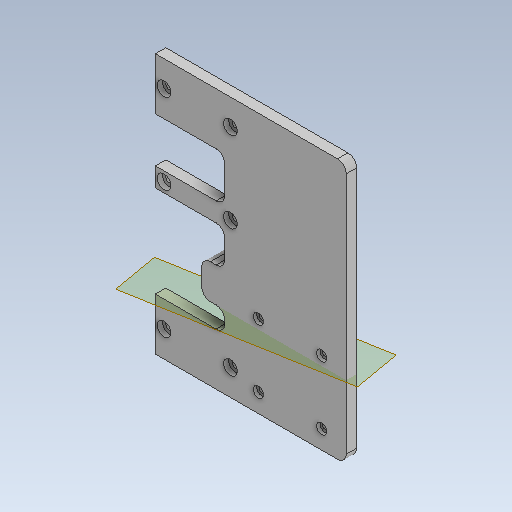
# Autodesk Inventor part: PlacaBase
Saved by Autodesk Inventor 2021 (Build 250183000, 183)
## iProperties
Created: 2022-10-28
Part Number: PlacaBase
Material: Generic
Document SubType Name: Modeling
Designer: zulet
Density: 1 g/cm^3
Appearance: Default
Author: zulet
Autodesk Inventor part; units mm, degrees
ref_plane "YZ Plane" through (0, 0, 0) normal (1, 0, 0) x (0, 1, 0)
ref_plane "XZ Plane" through (0, 0, 0) normal (0, 1, 0) x (-1, 0, 0)
ref_plane "XY Plane" through (0, 0, 0) normal (0, 0, 1) x (1, 0, 0)
sketch "Sketch1" plane through (0, 0, 0) normal (0, 0, 1) x (1, 0, 0)
  line L0 (-40, -150) -> (70, -150)
  line L1 (70, -150) -> (70, 0)
  line L2 (70, 0) -> (-40, 0)
  line L3 (-40, 0) -> (-40, -30)
  line L4 (-40, -30) -> (0, -30)
  line L5 (0, -30) -> (0, -56)
  line L6 (0, -56) -> (-40, -56)
  line L7 (-40, -56) -> (-40, -67)
  line L8 (-40, -67) -> (0, -67)
  line L9 (0, -67) -> (0, -120)
  line L10 (0, -120) -> (-40, -120)
  line L11 (-40, -120) -> (-40, -150)
  circle A0 centre (-35, -15) radius 2
  circle A1 centre (3.24, -15) radius 2
  line L12 (-35, -15) -> (3.24, -15) construction
  line L13 (-35, -15) -> (-40, -15) construction
  line L14 (-62, 0) -> (92, 0) projected
  line L15 (0, -180) -> (0, 30) projected
  circle A2 centre (-35, -61.5) radius 2
  circle A3 centre (3.24, -61.5) radius 2
  line L16 (-35, -61.5) -> (3.24, -61.5) construction
  circle A4 centre (-35, -135) radius 2
  line L17 (-35, -135) -> (3.24, -135) construction
  circle A5 centre (3.24, -135) radius 2
  line L18 (9.12, -7) -> (66.12, -7)
  line L19 (66.12, -7) -> (66.12, -92)
  line L20 (66.12, -92) -> (9.12, -92)
  line L21 (9.12, -92) -> (9.12, -7)
  line L22 (15.62, -99) -> (59.62, -99)
  line L23 (59.62, -99) -> (59.62, -143)
  line L24 (59.62, -143) -> (15.62, -143)
  line L25 (15.62, -143) -> (15.62, -99)
  line L26 (15.62, -99) -> (59.62, -143) construction
  line L27 (15.62, -143) -> (59.62, -99) construction
  circle A6 centre (19.37, -102.75) radius 1.5
  circle A7 centre (19.37, -139.25) radius 1.5
  circle A8 centre (55.87, -139.25) radius 1.5
  circle A9 centre (55.87, -102.75) radius 1.5
  line L28 (19.37, -102.75) -> (19.37, -139.25) construction
  line L29 (19.37, -139.25) -> (55.87, -139.25) construction
  line L30 (55.87, -139.25) -> (55.87, -102.75) construction
  line L31 (55.87, -102.75) -> (19.37, -102.75) construction
  line L32 (37.62, -7) -> (37.62, -92) construction
  line L33 (37.62, -99) -> (37.62, -143) construction
  point P0 (0, 0)
  dimension "d2" = 4
  dimension "d3" = 4
  dimension "d4" = 38.24
  dimension "d5" = 5
  dimension "d6" = 30
  dimension "d7" = 11
  dimension "d8" = 30
  dimension "d11" = 46.5
  dimension "d18" = 46.5
  dimension "d25" = 120
  dimension "d30" = 57
  dimension "d31" = 85
  dimension "d32" = 44
  dimension "d33" = 44
  dimension "d34" = 40
  dimension "d35" = 70
  dimension "d36" = 3
  dimension "d37" = 3
  dimension "d38" = 3
  dimension "d39" = 3
  dimension "d40" = 36.5
  dimension "d42" = 7
  dimension "d43" = 7
  dimension "d44" = 7
  dimension "d45" = 3.88
  dimension "d46" = 3.88
  constraints: 64 end point, 13 perpendicular, 10 centre point, 9 point on line, 6 horizontal, 5 midpoint, 4 collinear, 4 parallel, 4 vertical, 14 other
  measures "d2" diameter of A0
  measures "d3" diameter of A1
  measures "d4" distance of L12.start L12.end
  measures "d5" distance of L12.start L13.end
  measures "d6" distance between parallel lines of L4 L2
  measures "d7" distance between parallel lines of L8 L6
  measures "d8" distance between parallel lines of L0 L10
  measures "d11" distance of L12.start A2.centre
  measures "d18" distance of L12.start L16.start
  measures "d25" distance of L12.start L17.start
  measures "d30" distance of L19.end L20.end
  measures "d31" distance of L18.end L19.end
  measures "d32" distance of L23.end L24.end
  measures "d33" distance of L22.end L23.end
  measures "d34" distance between parallel lines of L15 L3
  measures "d35" distance between parallel lines of L1 L15
  measures "d36" diameter of A6
  measures "d37" diameter of A7
  measures "d38" diameter of A8
  measures "d39" diameter of A9
  measures "d40" distance of L28.end L28.start
  measures "d42" distance between parallel lines of L18 L14
  measures "d43" distance between parallel lines of L22 L20
  measures "d44" distance between parallel lines of L0 L24
  measures "d45" distance edge to line of A3 L21
  measures "d46" distance between parallel lines of L1 L19
extrude "Extrusion1" add sketch "Sketch1" along normal blind 6 contours L11 L10 L15 L0 | L15 L9 L5 L2 L1 L0 | L8 L7 L6 L15 | L15 L4 L3 L2
sketch "Sketch2" plane through (0, 0, 6) normal (0, 0, 1) x (1, 0, 0)
  line L0 (0, -56) -> (-40, -56) projected
  line L1 (-40, -56) -> (-40, -67) projected
  line L2 (-40, -67) -> (0, -67) projected
  line L3 (0, -67) -> (0, -120) projected
  line L4 (0, -120) -> (-40, -120) projected
  line L5 (-40, -120) -> (-40, -150) projected
  line L6 (-40, -150) -> (70, -150) projected
  line L7 (70, -150) -> (70, 0) projected
  line L8 (70, 0) -> (-40, 0) projected
  line L9 (-40, 0) -> (-40, -30) projected
  line L10 (-40, -30) -> (0, -30) projected
  line L11 (0, -30) -> (0, -56) projected
  circle A0 centre (-35, -15) radius 2 projected
  circle A1 centre (-35, -61.5) radius 2 projected
  circle A2 centre (-35, -135) radius 2 projected
  circle A3 centre (3.24, -15) radius 2 projected
  circle A4 centre (3.24, -61.5) radius 2 projected
  circle A5 centre (3.24, -135) radius 2 projected
  line L12 (15.62, -99) -> (59.62, -99) projected
  line L13 (59.62, -99) -> (59.62, -143) projected
  line L14 (59.62, -143) -> (15.62, -143) projected
  line L15 (15.62, -143) -> (15.62, -99) projected
  line L16 (9.12, -7) -> (66.12, -7) projected
  line L17 (66.12, -7) -> (66.12, -92) projected
  line L18 (66.12, -92) -> (9.12, -92) projected
  line L19 (9.12, -92) -> (9.12, -7) projected
  circle A6 centre (19.37, -102.75) radius 1.5 projected
  circle A7 centre (19.37, -139.25) radius 1.5 projected
  circle A8 centre (55.87, -139.25) radius 1.5 projected
  circle A9 centre (55.87, -102.75) radius 1.5 projected
  point P0 (0, 0)
extrude "Extrusion2" add sketch "Sketch2" against normal blind 3 contours L12 L13 L14 L15 | L16 L17 L18 L19
fillet "Fillet1" radius 5 6 edges at (0, -56, 3) (0, -30, 3) (0, -67, 3) (0, -120, 3) (70, 0, 3) (70, -150, 3)
sketch "Sketch3" plane through (0, 0, 6) normal (0, 0, 1) x (1, 0, 0)
  circle A0 centre (-35, -15) radius 2 projected
  circle A1 centre (-35, -15) radius 4
  circle A2 centre (3.24, -15) radius 2 projected
  circle A3 centre (3.24, -15) radius 4
  circle A4 centre (3.24, -61.5) radius 2 projected
  circle A5 centre (3.24, -61.5) radius 4
  circle A6 centre (-35, -61.5) radius 2 projected
  circle A7 centre (-35, -61.5) radius 4
  circle A8 centre (-35, -135) radius 2 projected
  circle A9 centre (-35, -135) radius 4
  circle A10 centre (3.24, -135) radius 2 projected
  circle A11 centre (3.24, -135) radius 4
  circle A12 centre (55.87, -102.75) radius 1.5 projected
  circle A13 centre (55.87, -102.75) radius 3
  circle A14 centre (55.87, -139.25) radius 1.5 projected
  circle A15 centre (55.87, -139.25) radius 3
  circle A16 centre (19.37, -139.25) radius 1.5 projected
  circle A17 centre (19.37, -139.25) radius 3
  circle A18 centre (19.37, -102.75) radius 1.5 projected
  circle A19 centre (19.37, -102.75) radius 3
  point P0 (0, 0)
  dimension "d50" = 8
  dimension "d51" = 8
  dimension "d52" = 8
  dimension "d53" = 8
  dimension "d54" = 8
  dimension "d55" = 8
  dimension "d58" = 6
  dimension "d59" = 6
  dimension "d60" = 6
  dimension "d61" = 6
  constraints: 10 centre point, 10 coincident
  measures "d50" diameter of A1
  measures "d51" diameter of A3
  measures "d52" diameter of A5
  measures "d53" diameter of A7
  measures "d54" diameter of A9
  measures "d55" diameter of A11
  measures "d58" diameter of A13
  measures "d59" diameter of A15
  measures "d60" diameter of A17
  measures "d61" diameter of A19
extrude "Extrusion3" cut sketch "Sketch3" against normal blind 3 contours A0 | A1 | A2 | A3 | A4 | A5 | A6 | A7 | A8 | A9 | A10 | A11
extrude "Extrusion4" cut sketch "Sketch3" against normal blind 2 contours A12 | A13 | A14 | A15 | A16 | A17 | A18 | A19
ref_plane "Work Plane1" through (-0.0065, -108, -32.8761) normal (0, -1, 0) x (-0.1736482, 0, -0.9848078)
sketch "Sketch5" plane through (-0.0065, -108, -32.8761) normal (0, -1, 0) x (-0.1736482, 0, -0.9848078)
  line L0 (-20, -17) -> (-20, 0) projected
  line L1 (-20, 0) -> (-32.9797, -2.2887)
  line L2 (-43.6649, 58.31) -> (-25.4318, -45.0948) projected
  line L3 (-25.4318, -45.0948) -> (-43.6649, 58.31) projected
  line L4 (-20, -17) -> (-35.9813, -19.8179)
  line L5 (-37.4183, -11.6684) -> (-31.3406, -46.1367) projected
  line L6 (-31.3406, -46.1367) -> (-49.5737, 57.2682) projected
  line L7 (-32.9797, -2.2887) -> (-38.8885, -3.3306)
  line L8 (-38.1546, -7.4928) -> (-39.5438, 0.3857) projected
  point P0 (-32.3777, -5.7025)
  constraints: 6 end point, 3 perpendicular, 3 point on line
extrude "Extrusion5" add sketch "Sketch5" against normal blind 20
fillet "Fillet2" radius 5 4 edges at (-13.2753, -88, -2.1139) (-13.2753, -108, -2.1139) (0, -88, 3) (0, -108, 3)
equation "\"d11\" = LMaSP"
equation "\"d18\" = LMaSP"
equation "\"d25\" = LM1aM2"
equation "\"d42\" = d44"
equation "\"d43\" = d42"
equation "\"d45\" = d46"
equation "\"d64\" = H1"
equation "\"H1\" = 20"
equation "\"DER\" = 22"
equation "\"HR\" = 7"
equation "\"DIR\" = 8"
equation "\"DEM\" = 4"
equation "\"Dmarc\" = 17.5"
equation "\"Bsm\" = 22.5"
equation "\"Hsm\" = 12"
equation "\"Lsm\" = 21"
equation "\"Dsc\" = 5"
equation "\"RC\" = 4"
equation "\"PB\" = 25"
equation "\"TB\" = 3"
equation "\"HSE\" = 25"
equation "\"LMaSP\" = 46.5"
equation "\"LM1aM2\" = 120"
body "Solid1"
